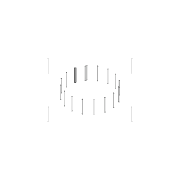
# Autodesk Inventor part: simple_ring5
Saved by Autodesk Inventor 2021 (Build 250183000, 183)
## iProperties
Created: 2022-04-11
Part Number: simple_ring5
Material: Generic
Document SubType Name: Modeling
Designer: Derm
Density: 1 g/cm^3
Appearance: Default
Author: Derm
Autodesk Inventor part; units mm, degrees
ref_plane "YZ Plane" through (0, 0, 0) normal (1, 0, 0) x (0, 1, 0)
ref_plane "XZ Plane" through (0, 0, 0) normal (0, 1, 0) x (-1, 0, 0)
ref_plane "XY Plane" through (0, 0, 0) normal (0, 0, 1) x (1, 0, 0)
sketch "Sketch1" plane through (0, 0, 0) normal (0, 1, 0) x (-1, 0, 0)
  circle A0 centre (0, 0) radius 5000 construction
  circle A1 centre (0, 0) radius 5000 construction
  circle A2 centre (0, 0) radius 5000 construction
  circle A3 centre (0, 0) radius 5000 construction
  circle A4 centre (0, 0) radius 5000 construction
  circle A5 centre (0, 0) radius 5000 construction
  circle A6 centre (0, 0) radius 5000 construction
  circle A7 centre (0, 0) radius 5000 construction
  circle A8 centre (0, 0) radius 5000 construction
  circle A9 centre (0, 0) radius 5000 construction
  circle A10 centre (0, 0) radius 5000 construction
  circle A11 centre (0, 0) radius 5000 construction
  circle A12 centre (0, 0) radius 5000 construction
  circle A13 centre (0, 0) radius 5000 construction
  circle A14 centre (0, 0) radius 5000 construction
  circle A15 centre (0, 0) radius 5000 construction
  ellipse E0 centre (4954.5587, 672.5686) end of major axis (5006.2311, 609.896) minor radius 59.6068
  ellipse E1 centre (2517.3999, -4320.0345) end of major axis (2333.7339, -4244.6033) minor radius 17.1666
  ellipse E2 centre (1274.6551, 4834.7962) end of major axis (1303.3021, 4850.8959) minor radius 195.7168
  ellipse E3 centre (-4320.0345, -2517.3999) end of major axis (-4137.1327, -2592.5171) minor radius 59.9346
  ellipse E4 centre (-2517.3999, 4320.0345) end of major axis (-2554.1884, 4230.4588) minor radius 95.611
  ellipse E5 centre (4320.0345, 2517.3999) end of major axis (4275.0482, 2517.3999) minor radius 108.5183
  ellipse E6 centre (3978.9799, -3027.8242) end of major axis (3988.3659, -3029.5312) minor radius 259.5498
  line L0 (4827.4649, -1111.3956) -> (4987.7998, -1217.2327)
  line L1 (4987.7998, -1217.2327) -> (4936.6889, -1402.4257)
  line L2 (4936.6889, -1402.4257) -> (4744.7658, -1411.0441)
  line L3 (4744.7658, -1411.0441) -> (4677.2616, -1231.1776)
  line L4 (4677.2616, -1231.1776) -> (4827.4649, -1111.3956)
  ellipse E7 centre (-4954.5587, -672.5686) end of major axis (-4890.2339, -760.2295) minor radius 81.2585
  circle A16 centre (10000, 0) radius 29.4088
  circle A17 centre (0, 10000) radius 29.4088
  circle A18 centre (-10000, 0) radius 29.4088
  circle A19 centre (0, -10000) radius 29.4088
  circle A20 centre (3027.8242, 3978.9799) radius 70.7666
  circle A21 centre (-3978.9799, 3027.8242) radius 55.0542
  circle A22 centre (672.5686, -4954.5587) radius 67.2342
  circle A23 centre (-1274.6551, -4834.7962) radius 52.8901
  circle A24 centre (-3027.8242, -3978.9799) radius 88.9601
  circle A25 centre (-4834.7962, 1274.6551) radius 100.4879
  ellipse E8 centre (-672.5686, 4954.5587) end of major axis (-648.729, 4844.36) minor radius 40.3117
  point P0 (4834.7962, -1274.6551)
  point P1 (4834.7962, -1274.6551)
  dimension "d0" = 10000
  dimension "d3" = 360
  dimension "d7" = 10000
  dimension "d10" = 360
  constraints: 19 coincident, 16 centre point, 10 end point, 123 other
  measures "d7" distance of point (0, 0) A16.centre
extrude "Extrusion1" add sketch "Sketch1" along normal mid plane 3000
body "Solid1"
